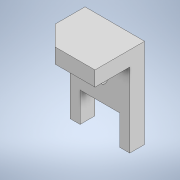
# Autodesk Inventor part: Ch3 Part 4
Saved by Autodesk Inventor 2020 (Build 240168000, 168)
## iProperties
Created: 2021-02-04
Part Number: Ch3 Part 4
Material: Generic
Document SubType Name: Modeling
Designer: austi
Density: 1 g/cm^3
Appearance: Default
Author: austi
Autodesk Inventor part; units mm, degrees
ref_plane "YZ Plane" through (0, 0, 0) normal (1, 0, 0) x (0, 1, 0)
ref_plane "XZ Plane" through (0, 0, 0) normal (0, 1, 0) x (-1, 0, 0)
ref_plane "XY Plane" through (0, 0, 0) normal (0, 0, 1) x (1, 0, 0)
sketch "Sketch1" plane through (0, 0, 0) normal (0, 0, 1) x (1, 0, 0)
  line L0 (0, 0) -> (0, 114.3)
  line L1 (0, 114.3) -> (76.2, 114.3)
  line L2 (76.2, 114.3) -> (76.2, 0)
  line L3 (76.2, 0) -> (63.5, 0)
  line L4 (63.5, 0) -> (63.5, 38.1)
  line L5 (63.5, 38.1) -> (12.7, 38.1)
  line L6 (12.7, 38.1) -> (12.7, 0)
  line L7 (12.7, 0) -> (0, 0)
  dimension "d0" = 114.3
  dimension "d1" = 76.2
  dimension "d2" = 12.7
  dimension "d3" = 38.1
  dimension "d4" = 50.8
  constraints: 16 end point, 7 perpendicular, 1 point on line, 1 vertical
  measures "d0" distance of L0.start L0.end
  measures "d1" distance of L0.end L1.end
  measures "d2" distance of L2.end L3.end
  measures "d3" distance of L3.end L4.end
  measures "d4" distance of L4.end L5.end
extrude "Extrusion1" add sketch "Sketch1" along normal blind 19.05
sketch "Sketch2" plane through (0, 0, 19.05) normal (0, 0, 1) x (1, 0, 0)
  line L0 (0, 114.3) -> (0, 0) projected
  line L1 (0, 114.3) -> (0, 95.25)
  line L2 (0, 95.25) -> (76.2, 95.25)
  line L3 (76.2, 0) -> (76.2, 114.3) projected
  line L4 (76.2, 95.25) -> (76.2, 114.3)
  line L5 (76.2, 114.3) -> (0, 114.3) projected
  line L6 (0, 114.3) -> (76.2, 114.3)
  dimension "d7" = 19.05
  constraints: 8 end point, 2 collinear, 2 point on line, 1 perpendicular
  measures "d7" distance of L0.start L1.end
extrude "Extrusion2" add sketch "Sketch2" along normal blind 44.45
chamfer "Chamfer1" distance 25.4 angle 45 1 edges at (0, 104.775, 63.5)
sketch "Sketch9" plane through (0, 0, 19.05) normal (0, 0, 1) x (1, 0, 0)
  circle A0 centre (38.1, 67.818) radius 9.525
  line L0 (63.5, 0) -> (76.2, 0) projected
  line L1 (0, 95.25) -> (0, 0) projected
  dimension "d15" = 19.05
  dimension "d16" = 67.818
  dimension "d17" = 38.1
  constraints: 1 centre point
  measures "d15" diameter of A0
  measures "d16" distance from line of A0.centre L0
  measures "d17" distance from line of A0.centre L1
hole "Hole1" at (38.1, 67.818, 19.05) direction (0, 0, -1) diameter 19.05 end through all
body "Solid1"
